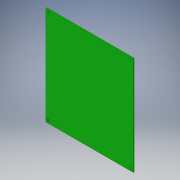
# Autodesk Inventor part: XGEN_simsun-pcb
Saved by Autodesk Inventor 2019 (Build 230136000, 136)
## iProperties
Created: 2019-02-28
Part Number: XGEN_simsun-pcb
Material: Generic
Document SubType Name: Sheet Metal
Designer: Rene
Density: 1 g/cm^3
Sheet Metal Rule: Default_mm
Appearance: Dark Green
Author: Rene
Autodesk Inventor part; units mm, degrees
ref_plane "YZ Plane" through (0, 0, 0) normal (1, 0, 0) x (0, 1, 0)
ref_plane "XZ Plane" through (0, 0, 0) normal (0, 1, 0) x (-1, 0, 0)
ref_plane "XY Plane" through (0, 0, 0) normal (0, 0, 1) x (1, 0, 0)
sketch "Sketch1" plane through (0, 0, 0) normal (0, 0, 1) x (1, 0, 0)
  line L0 (-80, -90) -> (80, -90)
  line L1 (80, -90) -> (80, 90)
  line L2 (-80, 90) -> (-80, -90)
  line L3 (32, 90) -> (32, 90)
  line L4 (32, 90) -> (-32, 90)
  line L5 (-32, 90) -> (-32, 90)
  line L6 (80, 90) -> (32, 90)
  line L7 (-32, 90) -> (-80, 90)
  point P0 (0, 0)
  dimension "d0" = 160
  dimension "d1" = 180
  dimension "d2" = 90
  dimension "d3" = 80
  dimension "d22" = 0
  dimension "d28" = 0
  dimension "d29" = 180
  constraints: 16 end point, 4 parallel, 1 horizontal, 1 perpendicular
  measures "d0" distance of L0.start L0.end
  measures "d1" distance of L2.start L0.start
  measures "d2" vertical distance of point (0, 0) L0.start
  measures "d3" horizontal distance of point (0, 0) L0.start
  measures "d22" distance of L4.end L5.end
  measures "d28" distance of L3.start L3.end
  measures "d29" distance of L0.end L1.end
extrude "Extrusion1" add sketch "Sketch1" along normal blind 2
sketch "Sketch2" plane through (0, 0, 2) normal (0, 0, 1) x (1, 0, 0)
  line L0 (-80, -90) -> (80, -90) projected
  line L1 (80, 90) -> (-80, 90) projected
  point P0 (0, 0)
  point P1 (-75, 85)
  point P2 (75, 85)
  point P3 (-75, -85)
  point P4 (75, -85)
  point P5 (-42, 105)
  point P6 (-80, 90)
  dimension "d6" = 170
  dimension "d8" = 150
  dimension "d9" = 75
  dimension "d10" = 150
  dimension "d11" = 5
  dimension "d12" = 5
  dimension "d13" = 170
  dimension "d14" = 75
  dimension "d27" = 5
  constraints: 1 other
  measures "d6" distance of point (-75, 85) point (-75, -85)
  measures "d8" distance of point (75, -85) point (-75, -85)
  measures "d9" horizontal distance of point (0, 0) point (-75, -85)
  measures "d10" distance of point (75, 85) point (-75, 85)
  measures "d11" distance from line of point (-75, -85) L0
  measures "d12" distance from line of point (75, -85) L0
  measures "d13" distance of point (75, 85) point (75, -85)
  measures "d14" horizontal distance of point (0, 0) point (-75, 85)
hole "Hole1" at (-75, 85, 2) at (75, 85, 2) at (-75, -85, 2) at (75, -85, 2) direction (0, 0, -1) diameter 4.2 end through all
equation "\"d2\" = 0.5 * d1"
equation "\"d3\" = 0.5 * d0"
equation "\"d29\" = d1"
equation "\"d9\" = 0.5 * d8"
equation "\"d10\" = d8"
equation "\"d12\" = d11"
equation "\"d13\" = d6"
equation "\"d14\" = d9"
equation "\"d20\" = Thickness"
equation "\"BendRadius\" = Thickness"
equation "\"BendReliefWidth\" = Thickness"
equation "\"BendReliefDepth\" = 0.5 * Thickness"
equation "\"CornerReliefSize\" = 4 * Thickness"
equation "\"MinimumRemnant\" = 2 * Thickness"
equation "\"TransitionRadius\" = BendRadius"
equation "\"JacobiRadiusSize\" = BendRadius"
equation "\"GapSize\" = Thickness"
equation "\"Thickness\" = 0.5"
body "Solid1"
